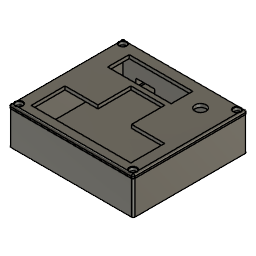
hackpadmodelv5 (Autodesk Fusion 360 design; units mm, degrees)
Autodesk Fusion 360 part; units mm, degrees
sketch "Sketch1" plane through (0, 0, 0) normal (0, 0, 1) x (1, 0, 0)
  line L0 (-90.4808, 59.85) -> (-28.0808, 59.85)
  line L1 (-28.0808, 59.85) -> (-28.0808, 3.45)
  line L2 (-28.0808, 3.45) -> (-90.4808, 3.45)
  line L3 (-90.4808, 3.45) -> (-90.4808, 59.85)
  dimension "d1" = 62.4
  dimension "d2" = 56.4
  constraint horizontal L0
  constraint vertical L1
  constraint horizontal L2
  constraint vertical L3
  measures "d1" distance of L0.start L0.end
  measures "d2" distance of L0.start L2.end
extrude "Extrude1" add sketch "Sketch1" along normal blind 14.6 makes body 1
shell "Shell1" thickness 5 outward yes removed faces 1 at (-69.6808, 41.05, 14.6) on bodies 1
ref_plane "WorkPlane1" through (-59.2808, 31.65, 14.6) normal (0, 0, 1) x (1, 0, 0)
sketch "Sketch2" plane through (0, 0, 14.6) normal (0, 0, 1) x (1, 0, 0)
  line L0 (-95.48, 64.8499) -> (-23.0806, 64.8499)
  line L1 (-23.0806, 64.8499) -> (-23.0806, -1.6501)
  line L2 (-23.0806, -1.6501) -> (-95.48, -1.6501)
  line L3 (-95.48, -1.6501) -> (-95.48, 64.8499)
  line L4 (-88.0462, 23.6829) -> (-30.0462, 23.6829)
  line L5 (-30.0462, 23.6829) -> (-30.0462, 4.0249)
  line L6 (-30.0462, 4.0249) -> (-88.0462, 4.0249)
  line L7 (-88.0462, 4.0249) -> (-88.0462, 23.6829)
  line L8 (-68.8631, 23.6829) -> (-49.2669, 23.6829)
  line L9 (-49.2669, 23.6829) -> (-49.2669, 42.9032)
  line L10 (-49.2669, 42.9032) -> (-68.8631, 42.9032)
  line L11 (-68.8631, 42.9032) -> (-68.8631, 23.6829)
  circle A0 centre (-37.446, 52.0157) radius 3.25
  line L12 (-85.1542, 58.1457) -> (-48.1542, 58.1457)
  line L13 (-48.1542, 58.1457) -> (-48.1542, 45.6457)
  line L14 (-48.1542, 45.6457) -> (-85.1542, 45.6457)
  line L15 (-85.1542, 45.6457) -> (-85.1542, 58.1457)
  dimension "d7" = 6.5
  dimension "d10" = 37
  dimension "d11" = 12.5
  dimension "d38" = 66.5
  constraint horizontal L0
  constraint vertical L1
  constraint horizontal L2
  constraint vertical L3
  constraint horizontal L4
  constraint vertical L5
  constraint horizontal L6
  constraint vertical L7
  constraint horizontal L8
  constraint vertical L9
  constraint horizontal L10
  constraint vertical L11
  constraint coincident L4 L8.start
  constraint horizontal L12
  constraint vertical L13
  constraint horizontal L14
  constraint vertical L15
  measures "d7" diameter of A0
  measures "d10" distance of L12.start L12.end
  measures "d11" distance of L12.start L14.end
  measures "d38" distance of L0.end L1.end
extrude "Extrude2" add sketch "Sketch2" along normal blind 2 separate body makes body 2
sketch "Sketch3" plane through (0, 0, 16.6) normal (0, 0, 1) x (-1, 0, 0)
  line L0 (49.2669, -42.9032) -> (49.2669, -23.6829)
  line L1 (49.2669, -23.6829) -> (30.0462, -23.6829)
  line L2 (30.0462, -23.6829) -> (30.0462, -4.0249)
  line L3 (30.0462, -4.0249) -> (88.0462, -4.0249)
  line L4 (88.0462, -4.0249) -> (88.0462, -23.6829)
  line L5 (88.0462, -23.6829) -> (68.8631, -23.6829)
  line L6 (68.8631, -23.6829) -> (68.8631, -42.9032)
  line L7 (68.8631, -42.9032) -> (49.2669, -42.9032)
  line L8 (48.1542, -45.6457) -> (85.1542, -45.6457)
  line L9 (85.1542, -45.6457) -> (85.1542, -58.1457)
  line L10 (85.1542, -58.1457) -> (48.1542, -58.1457)
  line L11 (48.1542, -58.1457) -> (48.1542, -45.6457)
  line L12 (95.48, 1.6501) -> (23.0806, 1.6501)
  line L13 (23.0806, 1.6501) -> (23.0806, -64.8499)
  line L14 (23.0806, -64.8499) -> (95.48, -64.8499)
  line L15 (95.48, -64.8499) -> (95.48, 1.6501)
  circle A0 centre (37.446, -52.0157) radius 3.25
sketch "Sketch4" plane through (0, 64.85, 0) normal (0, 1, 0) x (-1, 0, 0)
  line L0 (23.0808, -5) -> (95.4808, -5)
  line L1 (95.4808, -5) -> (95.4808, 14.6)
  line L2 (95.4808, 14.6) -> (23.0808, 14.6)
  line L3 (23.0808, 14.6) -> (23.0808, -5)
  line L4 (72, 0) -> (83, 0)
  line L5 (83, 0) -> (83, 4.9757)
  line L6 (83, 4.9757) -> (72, 4.9757)
  line L7 (72, 4.9757) -> (72, 0)
  constraint horizontal L4
  constraint vertical L5
  constraint horizontal L6
  constraint vertical L7
extrude "Extrude4" cut sketch "Sketch4" against normal blind 5 contours L4 L5 L6 L7 bodies 1
fillet "Fillet1" radius 1 4 edges at (-59.2803, -1.6501, 16.6) (-23.0806, 31.5999, 16.6) (-95.48, 31.5999, 16.6) (-59.2803, 64.8499, 16.6) on bodies 2
fillet "Fillet3" radius 1 12 edges at (-95.4808, -1.55, 4.8) (-23.0808, -1.55, 4.8) (-23.0808, 64.85, 4.8) (-95.4808, 64.85, 4.8) (-23.0806, -1.6501, 15.1) (-23.3735, -1.3572, 16.3071) (-95.48, -1.6501, 15.1) (-95.1871, -1.3572, 16.3071) (-23.3735, 64.557, 16.3071) (-23.0806, 64.8499, 15.1) (-95.1871, 64.557, 16.3071) (-95.48, 64.8499, 15.1) on bodies 1 2
fillet "Fillet3" radius 0.5 4 edges at (-72, 62.35, 0) (-72, 62.35, 4.9757) (-83, 62.35, 0) (-83, 62.35, 4.9757) on bodies 1 2
sketch "Sketch8" plane through (0, 0, 16.6) normal (0, 0, 1) x (-1, 0, 0)
  line L0 (94.48, 0.6501) -> (94.48, -63.8499)
  line L1 (94.48, -63.8499) -> (24.0806, -63.8499)
  circle A0 centre (92.48, -61.8499) radius 2
  line L2 (24.0806, 0.6501) -> (94.48, 0.6501)
  circle A1 centre (92.48, -1.3499) radius 2
  line L3 (24.0806, -63.8499) -> (24.0806, 0.6501)
  circle A2 centre (26.0806, -61.8499) radius 2
  circle A3 centre (26.0806, -1.3499) radius 2
  dimension "d39" = 2
  dimension "d40" = 2
  dimension "d41" = 2
  dimension "d42" = 2
  constraint tangent L0 A0
  constraint tangent L1 A0
  constraint tangent L0 A1
  constraint tangent L2 A1
  constraint tangent L1 A2
  constraint tangent L3 A2
  constraint tangent L3 A3
  constraint tangent L2 A3
  measures "d39" radius of A0
  measures "d40" radius of A1
  measures "d41" radius of A2
  measures "d42" radius of A3
extrude "Extrude6" cut sketch "Sketch8" against normal blind 5 contours A1 | A0 | A3 | A2 bodies 1 2
sketch "Sketch7" plane through (0, 0, 0) normal (0, 0, 1) x (-1, 0, 0)
  line L0 (82.5, -64.85) -> (82.5, -59.85)
  line L1 (82.5, -59.85) -> (90.4808, -59.85)
  line L2 (90.4808, -59.85) -> (90.4808, -3.45)
  line L3 (90.4808, -3.45) -> (28.0808, -3.45)
  line L4 (28.0808, -3.45) -> (28.0808, -59.85)
  line L5 (28.0808, -59.85) -> (72.5, -59.85)
  line L6 (72.5, -59.85) -> (72.5, -64.85)
  line L7 (72.5, -64.85) -> (82.5, -64.85)
  line L8 (28.0808, -59.85) -> (90.4808, -59.85)
  line L9 (90.4808, -59.85) -> (90.4808, -3.45)
  line L10 (90.4808, -3.45) -> (28.0808, -3.45)
  line L11 (28.0808, -3.45) -> (28.0808, -59.85)
  constraint horizontal L8
  constraint vertical L9
  constraint horizontal L10
  constraint vertical L11
  constraint coincident L2.end L3.start
  constraint coincident L4.end L5.start
fillet "Fillet4" radius 0.25 8 edges at (-91.0658, 60.4357, 16.6) (-93.8942, 63.2641, 16.6) (-91.0658, 2.7641, 16.6) (-93.8942, -0.0643, 16.6) (-27.4948, 2.7641, 16.6) (-24.6664, -0.0643, 16.6) (-27.4948, 60.4357, 16.6) (-24.6664, 63.2641, 16.6) on bodies 2
